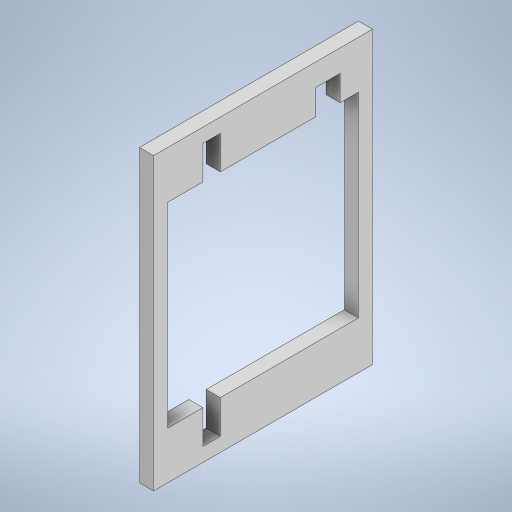
# Autodesk Inventor part: Part1
Saved by Autodesk Inventor 2023 (Build 270158000, 158)
## iProperties
Created: 2024-07-23
Part Number: Part1
Material: Generic
Document SubType Name: Modeling
Designer: Swoby
Density: 1 g/cm^3
Appearance: Default
Author: Swoby
Autodesk Inventor part; units mm, degrees
ref_plane "YZ Plane" through (0, 0, 0) normal (1, 0, 0) x (0, 1, 0)
ref_plane "XZ Plane" through (0, 0, 0) normal (0, 1, 0) x (-1, 0, 0)
ref_plane "XY Plane" through (0, 0, 0) normal (0, 0, 1) x (1, 0, 0)
sketch "Sketch1" plane through (0, 0, 0) normal (1, 0, 0) x (0, 1, 0)
  line L0 (0, 0) -> (-40.6, 0) construction
  line L1 (-40.6, -39.6) -> (0, -39.6) construction
  line L2 (0, -7.5) -> (7.1, -7.5) construction
  line L3 (7.1, -7.5) -> (7.1, -10.2) construction
  line L4 (7.1, -10.2) -> (0, -10.2) construction
  line L5 (0, -31.5) -> (5.4, -31.5) construction
  line L6 (5.4, -31.5) -> (5.4, -35.7) construction
  line L7 (5.4, -35.7) -> (0, -35.7) construction
  line L8 (-40.6, -7.5) -> (-47.7, -7.5) construction
  line L9 (-47.7, -7.5) -> (-47.7, -10.2) construction
  line L10 (-47.7, -10.2) -> (-40.6, -10.2) construction
  line L11 (0, -7.5) -> (0, 0) construction
  line L12 (0, -39.6) -> (0, -35.7) construction
  line L13 (0, -31.5) -> (0, -10.2) construction
  line L14 (-40.6, 0) -> (-40.6, -7.5) construction
  line L15 (-40.6, -10.2) -> (-40.6, -39.6) construction
  line L16 (-41.1, 0.5) -> (0.5, 0.5)
  line L17 (0.5, 0.5) -> (0.5, -7)
  line L18 (0.5, -7) -> (7.6, -7)
  line L19 (7.6, -7) -> (7.6, -10.7)
  line L20 (7.6, -10.7) -> (0.5, -10.7)
  line L21 (0.5, -10.7) -> (0.5, -31)
  line L22 (0.5, -31) -> (5.9, -31)
  line L23 (5.9, -31) -> (5.9, -36.2)
  line L24 (5.9, -36.2) -> (0.5, -36.2)
  line L25 (0.5, -36.2) -> (0.5, -40.1)
  line L26 (0.5, -40.1) -> (-41.1, -40.1)
  line L27 (-41.1, -40.1) -> (-41.1, -10.7)
  line L28 (-41.1, -10.7) -> (-48.2, -10.7)
  line L29 (-48.2, -10.7) -> (-48.2, -7)
  line L30 (-48.2, -7) -> (-41.1, -7)
  line L31 (-41.1, -7) -> (-41.1, 0.5)
  line L32 (10.6, 3.5) -> (-51.2, 3.5)
  line L33 (-51.2, 3.5) -> (-51.2, -43.1)
  line L34 (-51.2, -43.1) -> (10.6, -43.1)
  line L35 (10.6, -43.1) -> (10.6, 3.5)
  point P0 (7.6, -8.85)
  point P1 (-48.2, -8.85)
  dimension "d0" = 40.6
  dimension "d1" = 39.6
  dimension "d2" = 7.1
  dimension "d3" = 7.1
  dimension "d4" = 2.7
  dimension "d5" = 2.7
  dimension "d6" = 7.5
  dimension "d7" = 3.9
  dimension "d8" = 4.2
  dimension "d9" = 5.4
  dimension "d10" = 0.5
  dimension "d11" = 3
  dimension "d12" = 3
  dimension "d13" = 3
  dimension "d14" = 3
  constraints: 72 end point, 22 parallel, 11 perpendicular, 6 collinear, 5 horizontal, 2 midpoint, 1 coincident, 1 point on line, 15 other
  measures "d0" distance of L0.start L0.end
  measures "d1" distance between parallel lines of L1 L0
  measures "d2" distance of L2.start L2.end
  measures "d3" distance of L8.start L8.end
  measures "d4" distance of L2.end L3.end
  measures "d5" distance of L8.end L9.end
  measures "d6" distance between parallel lines of L8 L0
  measures "d7" distance between parallel lines of L1 L7
  measures "d8" distance of L5.end L6.end
  measures "d9" distance between parallel lines of L13 L6
  measures "d10" distance between parallel lines of L0 L16
  measures "d11" distance from line of L35 point (7.6, -8.85)
  measures "d12" distance between parallel lines of L32 L16
  measures "d13" distance from line of L33 point (-48.2, -8.85)
  measures "d14" distance between parallel lines of L34 L26
extrude "Extrusion1" add sketch "Sketch1" along normal blind 3
body "Solid1"
